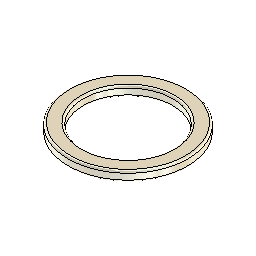
12-9x1 (Autodesk Fusion 360 design; units mm, degrees)
Autodesk Fusion 360 part; units mm, degrees
sketch "Sketch1" plane through (0, 0, 0) normal (0, 0, 1) x (1, 0, 0)
  circle A0 centre (0, 0) radius 4.5
  circle A1 centre (0, 0) radius 6
  dimension "d1" = 9
  dimension "d2" = 12
  constraint coincident A0.centre A1.centre
  measures "d1" diameter of A0
  measures "d2" diameter of A1
extrude "Extrude1" add sketch "Sketch1" along normal blind 1
fillet "Fillet1" radius 0.2 4 edges at (-5.594, -2.1697, 1) (-4.1955, 1.6273, 1) (-4.1955, 1.6273, 0) (-5.594, -2.1697, 0)
named bodies: "12-9x1"
